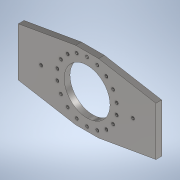
# Autodesk Inventor part: ODSY-0007-002
Saved by Autodesk Inventor 2021 (Build 250183000, 183)
## iProperties
Company: ERPL
Created: 2021-09-11
Material: Stainless Steel
Document SubType Name: Modeling
Designer: ALEX CLAY
Density: 8 g/cm^3
Appearance: Semi-Polished
Mass: 3249.37 g
Surface Area: 839.909 cm^2
Volume: 406.171 cm^3
Project: ODYSSEY
Description: ODYSSEY ENGINE MOUNT
Part Number: ODSY-0007-002
Author: ALEX CLAY
Revision Number: 00
Autodesk Inventor part; units mm, degrees
ref_plane "YZ Plane" through (0, 0, 0) normal (1, 0, 0) x (0, 1, 0)
ref_plane "XZ Plane" through (0, 0, 0) normal (0, 1, 0) x (-1, 0, 0)
ref_plane "XY Plane" through (0, 0, 0) normal (0, 0, 1) x (1, 0, 0)
sketch "Sketch1" plane through (0, 0, 0) normal (0, 0, 1) x (1, 0, 0)
  line L0 (-152.4, 53.975) -> (-152.4, -53.975)
  line L1 (-152.4, -53.975) -> (-25.4, -76.2)
  line L2 (-25.4, -76.2) -> (25.4, -76.2)
  line L3 (25.4, -76.2) -> (152.4, -53.975)
  line L4 (152.4, -53.975) -> (152.4, 53.975)
  line L5 (152.4, 53.975) -> (25.4, 76.2)
  line L6 (25.4, 76.2) -> (-25.4, 76.2)
  line L7 (-25.4, 76.2) -> (-152.4, 53.975)
  point P0 (0, 0)
  dimension "d59" = 152.4
  dimension "d60" = 304.8
  dimension "d61" = 76.2
  dimension "d62" = 152.4
  dimension "d64" = 50.8
  dimension "d65" = 25.4
  dimension "d66" = 107.95
  constraints: 16 end point, 2 horizontal alignment, 2 parallel, 2 vertical alignment, 1 horizontal, 1 perpendicular, 1 vertical
  measures "d59" distance between parallel lines of L2 L6
  measures "d60" distance between parallel lines of L4 L0
  measures "d61" distance from line of point (0, 0) L6
  measures "d62" distance from line of point (0, 0) L0
  measures "d64" distance of L5.end L6.end
  measures "d65" horizontal distance of point (0, 0) L6.end
  measures "d66" distance of L0.start L0.end
extrude "Extrusion1" add sketch "Sketch1" along normal mid plane 12.7
sketch "Sketch2" plane through (0, 0, 6.35) normal (0, 0, 1) x (1, 0, 0)
  circle A0 centre (0, 0) radius 50.8
  dimension "d4" = 101.6
  constraints: 1 centre point, 1 coincident
  measures "d4" diameter of A0
extrude "Extrusion2" cut sketch "Sketch2" against normal through all
sketch "Sketch5" plane through (0, 0, 6.35) normal (0, 0, 1) x (1, 0, 0)
  circle A0 centre (0, 0) radius 66.675 construction
  point P0 (0, 66.675)
  dimension "d36" = 133.35
  constraints: 2 vertical alignment, 1 coincident, 2 other
hole "Hole1" at (0, 66.675, 6.35) direction (0, 0, -1) diameter 6.7564 end through all clearance for "Flat Head Machine Screw (82)" size "1/4" standard "Ansi Unified Screw Threads"
pattern_circular "Circular Pattern1" count 18 over 360 about axis through (0, 0, 6.35) along (0, 0, -1) of "Hole1"
sketch "Sketch6" plane through (0, 0, -6.35) normal (0, 0, -1) x (-1, 0, 0)
  point P0 (0, 0)
  point P1 (-101.6, 0)
  point P2 (101.6, 0)
  dimension "d47" = 203.2
  dimension "d48" = 101.6
  constraints: 2 horizontal alignment
  measures "d47" distance of point (101.6, 0) point (-101.6, 0)
  measures "d48" distance of point (0, 0) point (-101.6, 0)
hole "Hole2" at (101.6, 0, -6.35) at (-101.6, 0, -6.35) direction (0, 0, 1) diameter 6.7564 end through all clearance for "Socket Head Cap Screw" size "1/4" standard "Ansi Unified Screw Threads"
equation "\"d61\" = 0.5 * d59"
equation "\"d62\" = 0.5 * d60"
equation "\"d65\" = 0.5 * d64"
body "Solid1"
